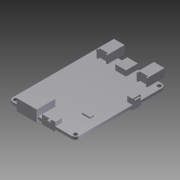
# Autodesk Inventor part: lipoRiderPro
Saved by Autodesk Inventor 2013 (Build 170138000, 138)
## iProperties
Created: 2012-12-27
Part Number: lipoRiderPro
Material: Generic
Document SubType Name: Modeling
Designer: otrebor
Density: 1 g/cm^3
Author: otrebor
Autodesk Inventor part; units mm, degrees
ref_plane "YZ Plane" through (0, 0, 0) normal (1, 0, 0) x (0, 1, 0)
ref_plane "XZ Plane" through (0, 0, 0) normal (0, 1, 0) x (-1, 0, 0)
ref_plane "XY Plane" through (0, 0, 0) normal (0, 0, 1) x (1, 0, 0)
sketch "Boceto1" plane through (0, 0, 0) normal (0, 0, 1) x (1, 0, 0)
  line L0 (0, 0) -> (50, 0)
  line L1 (50, 0) -> (50, 68)
  line L2 (50, 68) -> (0, 68)
  line L3 (0, 68) -> (0, 0)
  dimension "d0" = 50
  dimension "d1" = 68
  constraints: 8 end point, 3 perpendicular, 1 horizontal
  measures "d0" distance of L0.start L0.end
  measures "d1" distance of L0.end L1.end
extrude "Extrusión1" add sketch "Boceto1" along normal blind 2
hole "Hole1" at (2.0897, 65.5, 2) direction (0, 0, -1) diameter 3 end through all
hole "Hole2" at (47.5, 65.5, 2) direction (0, 0, -1) diameter 3 end through all
hole "Hole3" at (2.5, 2.5, 2) direction (0, 0, -1) diameter 3 end through all
hole "Hole4" at (47.5, 2.5, 2) direction (0, 0, -1) diameter 3 end through all
fillet "Empalme1" radius 3 1 edges at (50, 68, 1)
fillet "Empalme2" radius 3 1 edges at (0, 68, 1)
fillet "Empalme3" radius 3 1 edges at (0, 0, 1)
fillet "Empalme4" radius 3 1 edges at (50, 0, 1)
sketch "Boceto2" plane through (0, 0, 2) normal (0, 0, 1) x (1, 0, 0)
  line L0 (3, 68) -> (47, 68) projected
  line L1 (6, 68) -> (6, 60)
  line L2 (6, 60) -> (14, 60)
  line L3 (14, 60) -> (14, 68)
  line L4 (47, 0) -> (3, 0) projected
  line L5 (6, 68) -> (6, 73)
  line L6 (6, 73) -> (14, 73)
  line L7 (14, 73) -> (14, 68)
  point P0 (0, 0)
  dimension "d47" = 8
  dimension "d48" = 8
  dimension "d49" = 8
  dimension "d63" = 5
  constraints: 12 end point, 4 perpendicular, 1 collinear, 1 parallel, 1 point on line
  measures "d47" distance of L1.start L1.end
  measures "d48" distance of L1.end L2.end
  measures "d49" distance of L2.end L3.end
  measures "d63" distance of L1.start L5.end
extrude "Extrusión2" add sketch "Boceto2" along normal blind 6
sketch "Boceto3" plane through (0, 0, 8) normal (0, 0, 1) x (1, 0, 0)
  line L0 (6, 60) -> (6, 73) projected
  line L1 (14, 60) -> (6, 60) projected
  line L2 (14, 73) -> (14, 60) projected
  line L3 (6, 60) -> (7, 60)
  line L4 (7, 61.5) -> (6, 61.5)
  line L5 (7, 61.5) -> (7, 60)
  line L6 (14, 60) -> (13, 60)
  line L7 (13, 61.5) -> (14, 61.5)
  line L8 (13, 61.5) -> (13, 60)
  line L9 (7, 61.5) -> (13, 61.5)
  point P0 (14, 68)
  point P1 (6, 68)
  point P2 (0, 0)
  constraints: 14 end point, 5 perpendicular, 4 point on line
extrude "Extrusión3" cut sketch "Boceto3" against normal blind 6 contours L5 L9 L8 L1
sketch "Boceto4" plane through (0, 0, 2) normal (0, 0, 1) x (1, 0, 0)
  line L0 (14, 68) -> (14, 60) projected
  line L1 (6, 60) -> (6, 68) projected
  line L2 (3, 68) -> (47, 68) projected
  line L3 (6, 68) -> (14, 68)
  line L4 (21, 68) -> (21, 59)
  line L5 (21, 59) -> (29, 59)
  line L6 (29, 59) -> (29, 68)
  line L7 (21, 68) -> (29, 68)
  point P0 (0, 0)
  dimension "d55" = 8
  constraints: 10 end point, 4 point on line, 3 perpendicular, 1 collinear
  measures "d55" distance of L4.end L5.end
extrude "Extrusión4" add sketch "Boceto4" along normal blind 4
sketch "Boceto5" plane through (0, 0, 2) normal (0, 0, 1) x (1, 0, 0)
  line L0 (29, 68) -> (47, 68) projected
  line L1 (50, 68) -> (44, 68)
  line L2 (44, 68) -> (44, 60)
  line L3 (44, 60) -> (36, 60)
  line L4 (36, 60) -> (36, 73)
  line L5 (44, 73) -> (44, 65.5)
  line L6 (44, 73) -> (36, 73)
  point P0 (0, 0)
  dimension "d58" = 6
  dimension "d59" = 8
  dimension "d60" = 13
  constraints: 12 end point, 3 perpendicular, 2 point on line, 1 parallel
  measures "d58" distance of L1.start L1.end
  measures "d59" distance of L2.end L3.end
  measures "d60" distance of L3.end L4.end
extrude "Extrusión5" add sketch "Boceto5" along normal blind 6
sketch "Boceto6" plane through (0, 0, 8) normal (0, 0, 1) x (1, 0, 0)
  line L0 (44, 60) -> (36, 60) projected
  line L1 (37, 61.5) -> (37, 60)
  line L2 (43, 61.5) -> (43, 60)
  line L3 (43, 61.5) -> (37, 61.5)
  line L4 (37, 61.5) -> (37, 60)
  line L5 (43, 60.1438) -> (43, 61.5)
  line L6 (37, 60) -> (43, 60)
  point P0 (0, 0)
  constraints: 12 end point, 3 collinear, 2 point on line, 1 perpendicular
extrude "Extrusión6" cut sketch "Boceto6" against normal blind 6
sketch "Boceto7" plane through (0, 0, 2) normal (0, 0, 1) x (1, 0, 0)
  line L0 (0, 3) -> (0, 65) projected
  line L1 (47, 0) -> (3, 0) projected
  line L2 (7, 0) -> (7, -1)
  line L3 (7, -1) -> (22, -1)
  line L4 (22, -1) -> (22, 13)
  line L5 (22, 13) -> (7, 13)
  line L6 (7, 13) -> (7, 0)
  point P0 (0, 0)
  constraints: 10 end point, 3 perpendicular, 1 point on line
extrude "Extrusión7" add sketch "Boceto7" along normal blind 5
sketch "Boceto8" plane through (0, 0, 2) normal (0, 0, 1) x (1, 0, 0)
  line L0 (47, 0) -> (22, 0) projected
  line L1 (35, 0) -> (35, 5)
  line L2 (35, 5) -> (25, 5)
  line L3 (25, 5) -> (25, 0)
  line L4 (35, 0) -> (25, 0)
  point P0 (0, 0)
  dimension "d74" = 5
  constraints: 8 end point, 3 perpendicular, 2 point on line, 1 parallel
  measures "d74" distance of L1.start L1.end
extrude "Extrusión8" add sketch "Boceto8" along normal blind 3
sketch "Boceto9" plane through (3, 0, 0) normal (0, -1, 0) x (1, 0, 0)
  line L0 (29, 5) -> (22, 5)
  line L1 (32, 5) -> (29, 5)
  line L2 (29, 5) -> (29, 3.7)
  line L3 (29, 3.7) -> (27.7, 3.7)
  line L4 (27.7, 3.7) -> (27.7, 5)
  line L5 (29, 5) -> (27.7, 5)
  point P0 (-3, 0)
  dimension "d78" = 1.3
  dimension "d79" = 1.3
  constraints: 12 end point, 2 perpendicular, 1 collinear, 1 parallel, 1 point on line
  measures "d78" distance of L0.start L2.end
  measures "d79" distance of L2.end L3.end
extrude "Extrusión9" add sketch "Boceto9" along normal blind 2
sketch "Boceto10" plane through (0, 0, 2) normal (0, 0, 1) x (1, 0, 0)
  line L0 (50, 65) -> (50, 3) projected
  line L1 (50, 49) -> (46, 49)
  line L2 (46, 49) -> (46, 43)
  line L3 (46, 43) -> (50, 43)
  line L4 (50, 49) -> (50, 43)
  point P0 (0, 0)
  dimension "d83" = 6
  constraints: 8 end point, 2 point on line, 1 collinear, 1 parallel, 1 perpendicular
  measures "d83" distance of L1.end L2.end
extrude "Extrusión10" add sketch "Boceto10" along normal blind 4
sketch "Boceto11" plane through (50, 65, 2) normal (1, 0, 0) x (0, 0, -1)
  line L0 (-3, -17) -> (-1, -17)
  line L1 (-1, -17) -> (-1, -21)
  line L2 (-1, -21) -> (-3, -21)
  line L3 (-3, -21) -> (-3, -17)
  point P0 (2, -65)
  constraints: 8 end point, 1 parallel
extrude "Extrusión11" add sketch "Boceto11" along normal blind 1
sketch "Boceto12" plane through (0, 0, 2) normal (0, 0, 1) x (1, 0, 0)
  line L0 (47, 0) -> (35, 0) projected
  line L1 (43, 18) -> (43, 21)
  line L2 (43, 21) -> (37, 21)
  line L3 (37, 21) -> (37, 18)
  line L4 (37, 18) -> (43, 18)
  point P0 (0, 0)
  dimension "d90" = 3
  dimension "d91" = 6
  constraints: 8 end point, 2 perpendicular, 1 parallel
  measures "d90" distance of L1.start L1.end
  measures "d91" distance of L1.end L2.end
extrude "Extrusión12" add sketch "Boceto12" along normal blind 1
sketch "Boceto13" plane through (0, 0, 5) normal (0, 0, 1) x (1, 0, 0)
  line L0 (35, 5) -> (35, 0) projected
  line L1 (30.7, 0) -> (25, 0) projected
  line L2 (32, 0) -> (32, -2) projected
  line L3 (25, 5) -> (35, 5)
  line L4 (35, 0) -> (25, 0)
  line L5 (25, 5) -> (25, 0)
  line L6 (35, 5) -> (35, 0)
  point P0 (0, 0)
  constraints: 8 end point, 2 collinear, 2 perpendicular
extrude "Extrusión13" add sketch "Boceto13" against normal blind 6.5
sketch "Boceto14" plane through (0, 0, 7) normal (0, 0, 1) x (1, 0, 0)
  line L0 (7, -1) -> (7, 13) projected
  line L1 (22, -1) -> (7, -1) projected
  line L2 (22, 13) -> (22, -1) projected
  line L3 (7, 13) -> (22, 13) projected
  line L4 (7, 13) -> (22, 13)
  line L5 (22, -1) -> (7, -1)
  point P0 (0, 0)
  constraints: 4 end point, 2 collinear
extrude "Extrusión14" add sketch "Boceto14" against normal blind 8.5
sketch "Boceto15" plane through (0, 0, 6) normal (0, 0, 1) x (1, 0, 0)
  line L0 (50, 49) -> (50, 43) projected
  line L1 (46, 49) -> (50, 49) projected
  line L2 (46, 49) -> (50, 49)
  line L3 (50, 43) -> (46, 43)
  line L4 (46, 43) -> (46, 49)
  point P0 (0, 0)
  constraints: 6 end point, 1 collinear, 1 perpendicular
extrude "Extrusión15" add sketch "Boceto15" against normal blind 7.5
